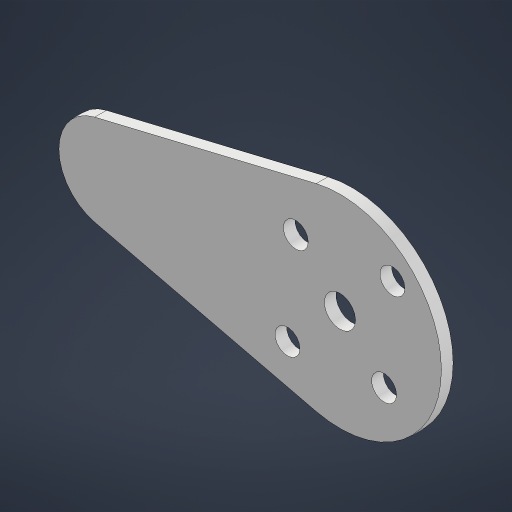
# Autodesk Inventor part: Dribler_main
Saved by Autodesk Inventor 2024.2 (Build 282272000, 272)
## iProperties
Created: 2023-12-22
Part Number: Dribler_main
Material: 一般
Document SubType Name: Modeling
Designer: Hanaoka
Density: 1 g/cm^3
Appearance: 既定
Author: Hanaoka
Autodesk Inventor part; units mm, degrees
ref_plane "YZ Plane" through (0, 0, 0) normal (1, 0, 0) x (0, 1, 0)
ref_plane "XZ Plane" through (0, 0, 0) normal (0, 1, 0) x (-1, 0, 0)
ref_plane "XY Plane" through (0, 0, 0) normal (0, 0, 1) x (1, 0, 0)
sketch "スケッチ1" plane through (0, 0, 0) normal (0, 0, 1) x (1, 0, 0)
  circle A0 centre (0, 0) radius 13
  line L0 (-3.0333, 12.6412) -> (-31.4, 5.8344)
  line L1 (-3.0333, -12.6412) -> (-31.4, -5.8344)
  arc A1 (-31.4, 5.8344) -> (-31.4, -5.8344) centre (-30, 0) ccw
  line L2 (-45.8, 0) -> (22.8, 0) projected
  circle A2 centre (-5.6569, 5.6569) radius 1.6 projected
  circle A3 centre (6.7175, 6.7175) radius 1.6 projected
  circle A4 centre (5.6569, -5.6569) radius 1.6 projected
  circle A5 centre (-6.7175, -6.7175) radius 1.6 projected
  circle A6 centre (0, 0) radius 2
  dimension "d0" = 30
  dimension "d1" = 26
  dimension "d2" = 6
  dimension "d5" = 4
  constraints: 4 end point, 4 point on circle, 4 tangent, 3 centre point, 2 coincident, 1 point on line
  measures "d0" distance of point (0, 0) A1.centre
  measures "d1" diameter of A0
  measures "d2" radius of A1
  measures "d5" diameter of A6
extrude "押し出し1" add sketch "スケッチ1" along normal blind 1.5 contours L2 A6 A0 | A0 L2 A6 | A0 L2 A1 L0 | L1 A1 L2 A0
